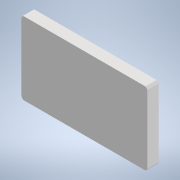
# Autodesk Inventor part: HDMI_Cover
Saved by Autodesk Inventor 2020 (Build 240168000, 168)
## iProperties
Created: 2020-08-08
Part Number: HDMI_Cover
Material: Generic
Document SubType Name: Modeling
Designer: reide
Density: 1 g/cm^3
Appearance: Default
Author: reide
Autodesk Inventor part; units mm, degrees
ref_plane "YZ Plane" through (0, 0, 0) normal (1, 0, 0) x (0, 1, 0)
ref_plane "XZ Plane" through (0, 0, 0) normal (0, 1, 0) x (-1, 0, 0)
sketch "Sketch1" plane through (0, 0, 0) normal (0, 0, 1) x (1, 0, 0)
  line L0 (18.75, 9.3095) -> (18.75, -2.6905) projected
  line L1 (-3.75, 9.8095) -> (18.25, 9.8095) projected
  line L2 (-4.25, -2.6905) -> (-4.25, 9.3095) projected
  line L3 (18.25, -3.1905) -> (-3.75, -3.1905) projected
  line L4 (-4, -3.1905) -> (18.5, -3.1905)
  line L5 (18.5, -3.1905) -> (18.5, 9.8095)
  line L6 (18.5, 9.8095) -> (-4, 9.8095)
  line L7 (-4, 9.8095) -> (-4, -3.1905)
  line L8 (-4, -3.1905) -> (18.5, 9.8095) construction
  line L9 (18.5, -3.1905) -> (-4, 9.8095) construction
  point P0 (0, 0)
  point P1 (7.25, 3.3095)
  dimension "d0" = 22.5
  constraints: 12 end point, 2 midpoint, 2 parallel, 2 perpendicular
  measures "d0" distance of L4.start L4.end
ref_plane "Work Plane1" through (-57.25, -12.6725, 2) normal (0, 0, 1) x (1, 0, 0)
extrude "Extrusion1" add sketch "Sketch1" along normal up to surface (2 mm away)
fillet "Fillet1" radius 0.5 4 edges at (18.5, 9.8095, 1) (18.5, -3.1905, 1) (-4, 9.8095, 1) (-4, -3.1905, 1)
fillet "Fillet2" radius 0.5 8 edges at (18.3536, 9.663, 2) (18.5, 3.3095, 2) (18.3536, -3.0441, 2) (7.25, -3.1905, 2) (-3.8536, -3.0441, 2) (-4, 3.3095, 2) (-3.8536, 9.663, 2) (7.25, 9.8095, 2)
body "Solid1"
